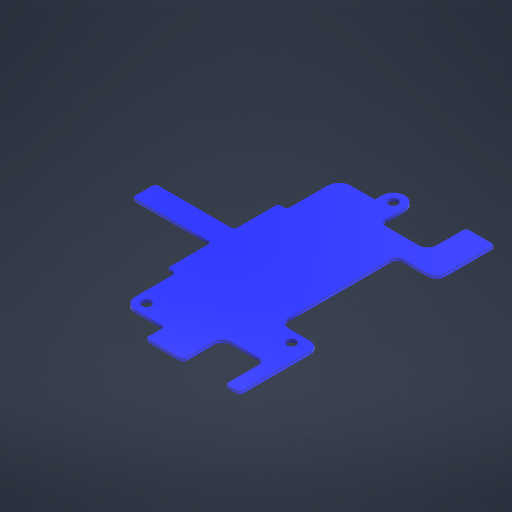
# Autodesk Inventor part: pcb
Saved by Autodesk Inventor 2024 (Build 280153000, 153)
## iProperties
Created: 2024-05-25
Part Number: pcb
Material: Generic
Document SubType Name: Modeling
Designer: Adam
Density: 1 g/cm^3
Appearance: Default
Author: Adam
Autodesk Inventor part; units mm, degrees
ref_plane "YZ Plane" through (0, 0, 0) normal (1, 0, 0) x (0, 1, 0)
ref_plane "XZ Plane" through (0, 0, 0) normal (0, 1, 0) x (-1, 0, 0)
ref_plane "XY Plane" through (0, 0, 0) normal (0, 0, 1) x (1, 0, 0)
ref_plane "Work Plane2" through (0, 1, 0) normal (0, 1, 0) x (1, 0, 0)
sketch "Sketch2" plane through (0, 1, 0) normal (0, 1, 0) x (1, 0, 0)
  line L0 (14.2983, 30.8418) -> (8.4694, 30.8418)
  line L1 (19.1771, -13.3933) -> (19.1771, 21.7206)
  line L2 (6.4694, 32.8418) -> (6.4694, 32.9551)
  line L3 (13.2983, -33.4026) -> (13.2983, -33.6636)
  arc A0 (-13.8229, -33.4026) -> (-9.8229, -37.4026) centre (-9.8229, -33.4026) ccw
  arc A1 (6.4694, 39.3998) -> (2.4699, 43.3408) centre (2.4699, 39.3408) ccw
  arc A2 (-9.8229, 36.9551) -> (-13.8229, 32.9551) centre (-9.8229, 32.9551) ccw
  arc A3 (6.4694, 32.8418) -> (8.4694, 30.8418) centre (8.4694, 32.8418) ccw
  circle A4 centre (2.4699, 39.3408) radius 1.55
  circle A5 centre (26.9336, -20.1907) radius 1.55
  circle A6 centre (-9.8229, -33.4026) radius 1.55
  line L4 (20.7089, 30.8418) -> (13.8839, 30.8418)
  line L5 (23.7927, 44.0538) -> (31.7927, 44.0538)
  line L6 (32.7927, 43.0538) -> (32.7927, 26.8418)
  line L7 (29.7927, 23.8418) -> (21.2983, 23.8418)
  line L8 (22.1771, -16.3933) -> (29.7927, -16.3933)
  line L9 (-17.8229, 3.7762) -> (-42.9549, 3.7762)
  line L10 (-43.9549, 2.7762) -> (-43.9549, -3.2238)
  line L11 (-42.9549, -4.2238) -> (-17.8229, -4.2238)
  arc A7 (15.8618, -30.3933) -> (13.2983, -33.4026) centre (16.3463, -33.4026) ccw
  line L12 (15.8618, -30.3933) -> (25.7927, -30.3933)
  line L13 (32.7927, -19.3933) -> (32.7927, -42.9467)
  line L14 (27.7927, -32.3933) -> (27.7927, -42.9467)
  line L15 (28.7927, -43.9467) -> (31.7927, -43.9467)
  line L16 (22.7927, 43.0538) -> (22.7927, 33.8418)
  line L17 (19.7927, 30.8418) -> (20.7089, 30.8418)
  arc A8 (23.7927, 44.0538) -> (22.7927, 43.0538) centre (23.7927, 43.0538) ccw
  arc A9 (32.7927, 43.0538) -> (31.7927, 44.0538) centre (31.7927, 43.0538) ccw
  arc A10 (31.7927, -43.9467) -> (32.7927, -42.9467) centre (31.7927, -42.9467) ccw
  arc A11 (27.7927, -42.9467) -> (28.7927, -43.9467) centre (28.7927, -42.9467) ccw
  arc A12 (29.7927, 23.8418) -> (32.7927, 26.8418) centre (29.7927, 26.8418) ccw
  arc A13 (19.7927, 30.8418) -> (22.7927, 33.8418) centre (19.7927, 33.8418) ccw
  arc A14 (27.7927, -32.3933) -> (25.7927, -30.3933) centre (25.7927, -32.3933) ccw
  arc A15 (19.1771, -13.3933) -> (22.1771, -16.3933) centre (22.1771, -13.3933) ccw
  arc A16 (32.7927, -19.3933) -> (29.7927, -16.3933) centre (29.7927, -19.3933) ccw
  arc A17 (21.2983, 23.8418) -> (19.1771, 21.7206) centre (21.2983, 21.7206) ccw
  arc A18 (-42.9549, 3.7762) -> (-43.9549, 2.7762) centre (-42.9549, 2.7762) ccw
  arc A19 (-43.9549, -3.2238) -> (-42.9549, -4.2238) centre (-42.9549, -3.2238) ccw
  line L18 (-13.8229, 32.9551) -> (-13.8229, 19.9551)
  line L19 (-14.8229, 18.9551) -> (-15.8229, 18.9551)
  line L20 (-16.8229, 17.9551) -> (-16.8229, 4.7762)
  line L21 (-13.8229, -33.4026) -> (-13.8229, -20.4026)
  line L22 (-14.8229, -19.4026) -> (-15.8229, -19.4026)
  line L23 (-16.8229, -18.4026) -> (-16.8229, -5.2238)
  arc A20 (-14.8229, 18.9551) -> (-13.8229, 19.9551) centre (-14.8229, 19.9551) ccw
  arc A21 (-15.8229, 18.9551) -> (-16.8229, 17.9551) centre (-15.8229, 17.9551) ccw
  arc A22 (-17.8229, 3.7762) -> (-16.8229, 4.7762) centre (-17.8229, 4.7762) ccw
  arc A23 (-16.8229, -5.2238) -> (-17.8229, -4.2238) centre (-17.8229, -5.2238) ccw
  arc A24 (-16.8229, -18.4026) -> (-15.8229, -19.4026) centre (-15.8229, -18.4026) ccw
  arc A25 (-13.8229, -20.4026) -> (-14.8229, -19.4026) centre (-14.8229, -20.4026) ccw
  line L24 (6.4694, 39.3998) -> (6.4694, 32.9551)
  arc A26 (2.4699, 43.3408) -> (-1.5298, 39.3918) centre (2.4699, 39.3408) ccw
  line L25 (-1.5298, 39.3918) -> (-1.5298, 36.9551)
  line L26 (-1.5298, 36.9551) -> (-9.8229, 36.9551)
  line L27 (13.2983, -33.4026) -> (13.2983, -42.9467)
  line L28 (12.2983, -43.9467) -> (1.2983, -43.9467)
  line L29 (0.2983, -42.9467) -> (0.2983, -38.4026)
  line L30 (-0.7017, -37.4026) -> (-9.8229, -37.4026)
  arc A27 (0.2983, -42.9467) -> (1.2983, -43.9467) centre (1.2983, -42.9467) ccw
  arc A28 (12.2983, -43.9467) -> (13.2983, -42.9467) centre (12.2983, -42.9467) ccw
  arc A29 (0.2983, -38.4026) -> (-0.7017, -37.4026) centre (-0.7017, -38.4026) ccw
  point P0 (0, 0)
  point P1 (19.1771, -27.6636)
  point P2 (13.2983, -31.6636)
  point P3 (19.1771, 23.8418)
  point P4 (22.7927, 44.0538)
  point P5 (32.7927, 44.0538)
  point P6 (32.7927, 23.8418)
  point P7 (32.7927, -16.3933)
  point P8 (32.7927, -43.9467)
  point P9 (27.7927, -30.3933)
  point P10 (25.9849, -16.3933)
  point P11 (19.1771, -16.3933)
  point P12 (-16.8229, 3.7762)
  point P13 (-16.8229, -4.2238)
  point P14 (30.2927, -43.9467)
  point P15 (-13.8229, 18.9551)
  point P16 (-16.8229, 18.9551)
  point P17 (-13.8229, -19.4026)
  point P18 (-16.8229, -19.4026)
  point P19 (13.2983, -43.9467)
  point P20 (0.2983, -43.9467)
  point P21 (0.2983, -37.4026)
  dimension "d12" = 2
  dimension "d13" = 3.1
  dimension "d15" = 3.1
  dimension "d19" = 7
  dimension "d23" = 5
  dimension "d24" = 10
  dimension "d26" = 1
  dimension "d27" = 3
  dimension "d28" = 2
  dimension "d30" = 3
  dimension "d32" = 1
  dimension "d33" = 20.212
  dimension "d35" = 14
  dimension "d36" = 14
  dimension "d37" = 3
  dimension "d38" = 14
  dimension "d39" = 3
  dimension "d40" = 1
  dimension "d41" = 36
  dimension "d42" = 13
  dimension "d43" = 1
  constraints: 62 end point, 54 point on circle, 46 tangent, 37 point on line, 30 centre point, 14 perpendicular, 13 equal radius, 8 vertical, 3 horizontal, 2 coincident, 2 midpoint, 1 parallel
  measures "d12" radius of A3
  measures "d13" diameter of A4
  measures "d15" diameter of A6
  measures "d19" distance between parallel lines of L7 L4
  measures "d23" distance between parallel lines of L13 L14
  measures "d24" distance between parallel lines of L6 L16
  measures "d26" radius of A8
  measures "d27" radius of A12
  measures "d28" radius of A14
  measures "d30" radius of A15
  measures "d32" radius of A18
  measures "d33" distance between parallel lines of L7 L5
  measures "d35" distance between parallel lines of L8 L12
  measures "d36" distance of L18.start point (-13.823, 18.955)
  measures "d37" distance of point (-13.823, 18.955) point (-16.823, 18.955)
  measures "d38" distance of L21.start point (-13.823, -19.403)
  measures "d39" distance between parallel lines of L21 L23
  measures "d40" radius of A20
  measures "d41" distance between parallel lines of L20 L1
  measures "d42" distance of point (13.298, -43.947) point (0.298, -43.947)
  measures "d43" radius of A27
extrude "Extrusion2" add sketch "Sketch2" along normal blind 1
body "Solid2"
